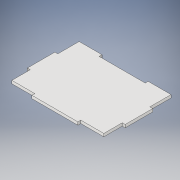
# Autodesk Inventor part: BASE_TAPA
Saved by Autodesk Inventor 2019 (Build 230136000, 136)
## iProperties
Created: 2020-02-12
Part Number: BASE_TAPA
Material: Genérico
Document SubType Name: Modeling
Designer: omar-
Density: 1 g/cm^3
Appearance: Valor por defecto
Author: omar-
Autodesk Inventor part; units mm, degrees
ref_plane "YZ Plane" through (0, 0, 0) normal (1, 0, 0) x (0, 1, 0)
ref_plane "XZ Plane" through (0, 0, 0) normal (0, 1, 0) x (-1, 0, 0)
ref_plane "XY Plane" through (0, 0, 0) normal (0, 0, 1) x (1, 0, 0)
sketch "Boceto1" plane through (0, 0, 0) normal (0, 1, 0) x (-1, 0, 0)
  line L0 (-50, -36.59) -> (50, -36.59)
  line L1 (50, -36.59) -> (50, 36.59)
  line L2 (50, 36.59) -> (-50, 36.59)
  line L3 (-50, 36.59) -> (-50, -36.59)
  line L4 (-50, -36.59) -> (50, 36.59) construction
  line L5 (50, -36.59) -> (-50, 36.59) construction
  line L6 (-19.9778, -36.59) -> (30.0222, -36.59)
  line L7 (-25, 39.77) -> (25, 39.77)
  line L8 (25, 39.77) -> (25, 36.59)
  line L9 (25, 36.59) -> (-25, 36.59)
  line L10 (-25, 36.59) -> (-25, 39.77)
  line L11 (-50, -13.41) -> (-50, 16.59)
  line L12 (53.18, 16.59) -> (50, 16.59)
  line L13 (50, 16.59) -> (50, -13.41)
  line L14 (50, -13.41) -> (53.18, -13.41)
  line L15 (53.18, -13.41) -> (53.18, 16.59)
  line L16 (-25, -33.41) -> (25, -33.41)
  line L17 (25, -33.41) -> (25, -36.59)
  line L18 (25, -36.59) -> (-25, -36.59)
  line L19 (-25, -36.59) -> (-25, -33.41)
  line L20 (-53.18, 16.59) -> (-50, 16.59)
  line L21 (-50, 16.59) -> (-50, -13.41)
  line L22 (-50, -13.41) -> (-53.18, -13.41)
  line L23 (-53.18, -13.41) -> (-53.18, 16.59)
  point P0 (0, 0)
  point P1 (0, 0)
  point P2 (0, 0)
  dimension "d0" = 100
  dimension "d1" = 73.18
  dimension "d2" = 3.18
  dimension "d3" = 50
  dimension "d4" = 25
  dimension "d6" = 30
  dimension "d8" = 20
  dimension "d10" = 50
  dimension "d11" = 25
  dimension "d16" = 3.18
  dimension "d17" = 20
  dimension "d18" = 30
  constraints: 48 end point, 10 parallel, 6 collinear, 6 horizontal, 5 perpendicular, 3 midpoint, 2 equal length, 1 coincident
  measures "d0" distance of L2.end L1.end
  measures "d1" distance of L0.end L1.end
  measures "d2" distance of L7.end L8.end
  measures "d3" distance of L7.start L7.end
  measures "d4" distance from line of point (0, 0) L8
  measures "d6" distance of L14.end L12.start
  measures "d8" distance between parallel lines of L2 L12
  measures "d10" distance of L16.start L16.end
  measures "d11" distance from line of L17 point (0, 0)
  measures "d16" distance of L12.start L12.end
  measures "d17" distance between parallel lines of L2 L20
  measures "d18" distance of L22.end L20.start
extrude "Extrusión1" add sketch "Boceto1" along normal blind 3.18 contours L3 L2 L1 L0 L17 L16 L19 | L22 L23 L20 L3 | L10 L7 L8 L2 | L1 L12 L15 L14
